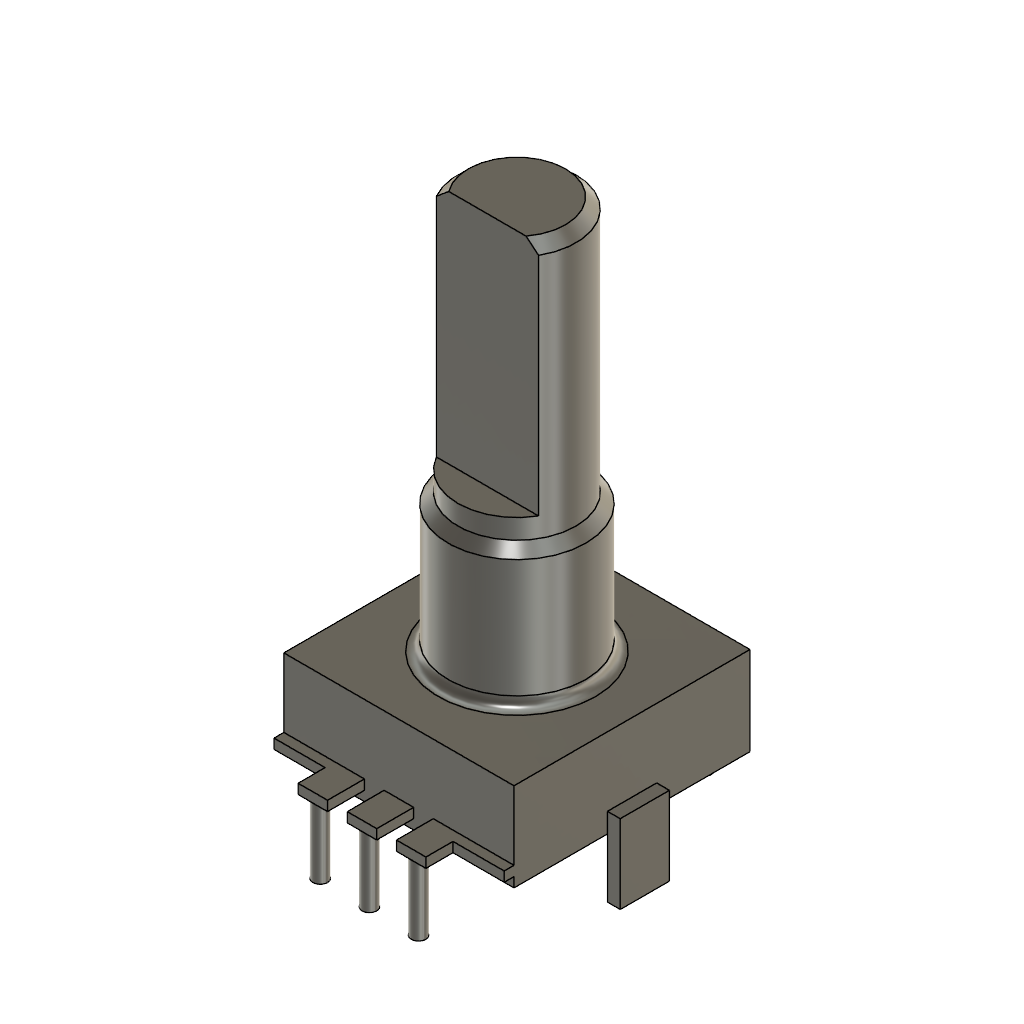
EC11E single rotary (Autodesk Fusion 360 design; units mm, degrees)
Autodesk Fusion 360 part; units mm, degrees
sketch "Skizze1" plane through (0, 0, 0) normal (0, 0, 1) x (1, 0, 0)
  line L0 (0, 0) -> (-11.7, 0)
  line L1 (-11.7, 0) -> (-11.7, 12)
  line L2 (-11.7, 12) -> (0, 12)
  line L3 (0, 12) -> (0, 0)
  dimension "d1" = 11.7
  dimension "d2" = 12
  constraint horizontal L0
  constraint vertical L1
  constraint horizontal L2
  constraint vertical L3
  constraint coincident L0.start L3.end
  measures "d1" distance of L1.end L2.end
  measures "d2" distance of L0.end L1.end
extrude "Extrusion1" add sketch "Skizze1" along normal blind 4.5
ref_plane "Arbeitsebene1" through (0, 0, 0.5) normal (0, 0, 1) x (1, 0, 0)
sketch "Skizze2" plane through (0, 0, 0.5) normal (0, 0, 1) x (1, 0, 0)
  line L0 (0, 12) -> (-11.7, 12)
  line L1 (-11.7, 12) -> (-11.7, 0)
  line L2 (-11.7, 0) -> (0, 0)
  line L3 (0, 0) -> (0, 12)
  line L4 (-8.35, 12) -> (-8.35, 19) construction
  line L5 (-3.35, 12) -> (-3.35, 19) construction
  line L6 (-8.35, 0) -> (-8.35, -5) construction
  line L7 (-5.85, 0) -> (-5.85, -5) construction
  line L8 (-3.35, 0) -> (-3.35, -5) construction
  line L9 (-7.6, 12) -> (-9.1, 12)
  line L10 (-9.1, 12) -> (-9.1, 13.375)
  line L11 (-9.1, 13.375) -> (-7.6, 13.375)
  line L12 (-7.6, 13.375) -> (-7.6, 12)
  line L13 (-2.6, 12) -> (-4.1, 12)
  line L14 (-4.1, 12) -> (-4.1, 13.375)
  line L15 (-4.1, 13.375) -> (-2.6, 13.375)
  line L16 (-2.6, 13.375) -> (-2.6, 12)
  line L17 (-2.6, 0) -> (-4.1, 0)
  line L18 (-4.1, 0) -> (-4.1, -1.875)
  line L19 (-4.1, -1.875) -> (-2.6, -1.875)
  line L20 (-2.6, -1.875) -> (-2.6, 0)
  line L21 (-6.6, 0) -> (-5.1, 0)
  line L22 (-5.1, 0) -> (-5.1, -1.875)
  line L23 (-5.1, -1.875) -> (-6.6, -1.875)
  line L24 (-6.6, -1.875) -> (-6.6, 0)
  line L25 (-9.1, 0) -> (-7.6, 0)
  line L26 (-7.6, 0) -> (-7.6, -1.875)
  line L27 (-7.6, -1.875) -> (-9.1, -1.875)
  line L28 (-9.1, -1.875) -> (-9.1, 0)
  line L29 (-9.1, 0) -> (-11.7, 0)
  line L30 (-11.7, 0) -> (-11.7, -0.5)
  line L31 (-11.7, -0.5) -> (-9.1, -0.5)
  line L32 (-9.1, -0.5) -> (-9.1, 0)
  line L33 (-2.6, 0) -> (0, 0)
  line L34 (0, 0) -> (0, -0.5)
  line L35 (0, -0.5) -> (-2.6, -0.5)
  line L36 (-2.6, -0.5) -> (-2.6, 0)
  circle A0 centre (-8.35, 13) radius 0.375
  circle A1 centre (-3.35, 13) radius 0.375
  circle A2 centre (-8.35, -1.5) radius 0.375
  circle A3 centre (-5.85, -1.5) radius 0.375
  circle A4 centre (-3.35, -1.5) radius 0.375
  line L37 (-11.7, 6) -> (0, 6) construction
  line L38 (-11.7, 7.25) -> (-12.35, 7.25)
  line L39 (-12.35, 7.25) -> (-12.35, 4.75)
  line L40 (-12.35, 4.75) -> (-11.7, 4.75)
  line L41 (-11.7, 4.75) -> (-11.7, 7.25)
  line L42 (0, 7.25) -> (0.65, 7.25)
  line L43 (0.65, 7.25) -> (0.65, 4.75)
  line L44 (0.65, 4.75) -> (0, 4.75)
  line L45 (0, 4.75) -> (0, 7.25)
  line L46 (-11.6, 7.25) -> (-11.6, 4.75)
  line L47 (-0.1, 7.25) -> (-0.1, 4.75)
  dimension "d7" = 5
  dimension "d8" = 5
  dimension "d9" = 1.5
  dimension "d11" = 0.5
  dimension "d12" = 0.75
  dimension "d13" = 0.75
  dimension "d14" = 0.75
  dimension "d15" = 0.75
  dimension "d16" = 0.75
  dimension "d17" = 7
  dimension "d18" = 7
  dimension "d19" = 7.5
  dimension "d20" = 7.5
  dimension "d21" = 7.5
  dimension "d26" = 0.75
  dimension "d27" = 0.75
  dimension "d28" = 13
  dimension "d46" = 2.5
  constraint coincident L0 L4.start
  constraint perpendicular L0 L4
  constraint coincident L0 L5.start
  constraint perpendicular L0 L5
  constraint coincident L2 L6.start
  constraint perpendicular L2 L6
  constraint midpoint L2 L7.start
  constraint perpendicular L2 L7
  constraint coincident L2 L8.start
  constraint perpendicular L2 L8
  constraint horizontal L9
  constraint vertical L10
  constraint horizontal L11
  constraint vertical L12
  constraint coincident L0 L9.start
  constraint horizontal L13
  constraint vertical L14
  constraint horizontal L15
  constraint vertical L16
  constraint coincident L0 L13.start
  constraint horizontal L17
  constraint vertical L18
  constraint horizontal L19
  constraint vertical L20
  constraint coincident L2 L17.start
  constraint horizontal L21
  constraint vertical L22
  constraint horizontal L23
  constraint vertical L24
  constraint coincident L2 L21.start
  constraint horizontal L25
  constraint vertical L26
  constraint horizontal L27
  constraint vertical L28
  constraint coincident L2 L25.start
  constraint symmetric L6.end L7 L8.end
  constraint symmetric L4.end L5.end L7
  constraint symmetric L4 L10 L12
  constraint symmetric L5 L14 L16
  constraint symmetric L7 L22 L24
  constraint equal L10 L14
  constraint equal L11 L15
  constraint equal L11 L27
  constraint equal L23 L27
  constraint equal L19 L23
  constraint horizontal L29
  constraint vertical L30
  constraint horizontal L31
  constraint vertical L32
  constraint horizontal L33
  constraint vertical L34
  constraint horizontal L35
  constraint vertical L36
  constraint equal L30 L34
  constraint coincident L1.end L2.start
  constraint coincident L4 A0.centre
  constraint coincident L5 A1.centre
  constraint coincident L6 A2.centre
  constraint coincident L7 A3.centre
  constraint coincident L8 A4.centre
  constraint midpoint L1 L37.start
  constraint midpoint L3 L37.end
  constraint tangent L11 A0
  constraint tangent L27 A2
  constraint tangent L23 A3
  constraint tangent L19 A4
  constraint horizontal L38
  constraint vertical L39
  constraint horizontal L40
  constraint vertical L41
  constraint coincident L1 L38.start
  constraint horizontal L42
  constraint vertical L43
  constraint horizontal L44
  constraint vertical L45
  constraint coincident L3 L42.start
  constraint symmetric L37 L38 L40
  constraint symmetric L37 L42 L44
  constraint equal L38 L42
  constraint equal L39 L43
  constraint coincident L38 L46.start
  constraint coincident L40 L46.end
  constraint perpendicular L40 L46
  constraint coincident L42 L47.start
  constraint coincident L44 L47.end
  constraint perpendicular L44 L47
  measures "d7" distance of L4 L5
  measures "d8" distance of L6 L8
  measures "d9" distance of L10.end L11.end
  measures "d11" distance of L1.end L30.end
  measures "d12" diameter of A0
  measures "d13" diameter of A1
  measures "d14" diameter of A2
  measures "d15" diameter of A3
  measures "d16" diameter of A4
  measures "d17" distance of A0.centre L37
  measures "d18" distance of A1.centre L37
  measures "d19" distance of A2.centre L37
  measures "d20" distance of A3.centre L37
  measures "d21" distance of A4.centre L37
  measures "d26" distance of L39 L46
  measures "d27" distance of L43 L47
  measures "d28" distance of L39 L43
  measures "d46" distance of L38.end L39.end
extrude "Extrusion2" add sketch "Skizze2" along normal blind 0.5 contours A1 | L0 L13 L14 L15 L16 | L3 L42 L43 L44 L45 | A0 | L0 L9 L10 L11 L12 | L2 L20 L33 L34 L35 L36 | A4 | L2 L17 L18 L19 L20 L36 | L1 L38 L39 L40 L41 | A3 | L2 L21 L22 L23 L24 | L2 L28 L29 L30 L31 L32 | A2 | L2 L25 L26 L27 L28 L32
extrude "Extrusion3" add sketch "Skizze2" against normal blind 3.5 contours A1 | L3 L42 L43 L44 L45 | A0 | A4 | L1 L38 L39 L40 L41 | A3 | A2
ref_plane "Arbeitsebene2" through (0, 6, 0) normal (0, 1, 0) x (0, 0, 1)
sketch "Skizze3" plane through (0, 6, 0) normal (0, 1, 0) x (1, 0, 0)
  line L0 (-4.1, -1) -> (0, -1)
  line L1 (0, -1) -> (0, -4.5)
  line L2 (0, -4.5) -> (-11.7, -4.5)
  line L3 (-11.7, -4.5) -> (-11.7, -1)
  line L4 (-11.7, -1) -> (-7.6, -1)
  line L5 (-7.6, -1) -> (-7.6, -0.5)
  line L6 (-7.6, -0.5) -> (-11.7, -0.5)
  line L7 (-11.7, -0.5) -> (-11.7, 0)
  line L8 (-11.7, 0) -> (0, 0)
  line L9 (0, 0) -> (0, -0.5)
  line L10 (0, -0.5) -> (-4.1, -0.5)
  line L11 (-4.1, -0.5) -> (-4.1, -1)
  line L12 (-5.1, -1) -> (-5.1, -0.5)
  line L13 (-5.1, -0.5) -> (-6.6, -0.5)
  line L14 (-6.6, -0.5) -> (-6.6, -1)
  line L15 (-6.6, -1) -> (-5.1, -1)
  line L16 (-5.85, -4.5) -> (-5.85, -18.5)
  line L17 (-5.85, -4.5) -> (-1.85, -4.5)
  line L18 (-2.35, -5) -> (-2.35, -11)
  arc A0 (-1.85, -4.5) -> (-2.35, -5) centre (-1.85, -5) ccw
  line L19 (-2.35, -11) -> (-2.85, -11.5)
  line L20 (-2.85, -11.5) -> (-2.85, -23.9697)
  line L21 (-2.85, -23.9697) -> (-3.3803, -24.5)
  line L22 (-3.3803, -24.5) -> (-5.85, -24.5)
  line L23 (-5.85, -24.5) -> (-5.85, -4.5)
  dimension "d31" = 1
  dimension "d32" = 7
  dimension "d33" = 6
  dimension "d34" = 135
  dimension "d35" = 135
  dimension "d36" = 7
  dimension "d40" = 0.75
  dimension "d41" = 20
  constraint midpoint L2 L16.start
  constraint perpendicular L2 L16
  constraint tangent L17 A0
  constraint vertical L18
  constraint tangent L18 A0
  constraint parallel L18 L20
  constraint coincident L16 L22.end
  constraint perpendicular L16 L22
  constraint horizontal L17
  measures "d31" diameter of A0
  measures "d34" angle of L18 L19
  measures "d35" angle of L20 L21
  measures "d36" distance of L17 L19.end
  measures "d40" distance of L20.end L21.end
  measures "d41" distance of L2 L22
revolve "Drehen1" add sketch "Skizze3" angle 360 about axis through (-5.85, 6, 4.5) along (0, 0, 1) contours L2 L16 L17 L18 A0 L19 L20 L21 L22 L23
sketch "Skizze4" plane through (0, 0, 24.5) normal (0, 0, 1) x (-1, 0, 0)
  circle A0 centre (5.85, -6) radius 2.4697
  circle A1 centre (5.85, -6) radius 3
  line L0 (8.4481, -4.5) -> (3.2519, -4.5)
  arc A2 (8.4481, -4.5) -> (3.2519, -4.5) centre (5.85, -6) ccw
  line L1 (5.85, -4.5) -> (5.85, -9) construction
  dimension "d43" = 4.5
  constraint coincident A1 L0.start
  constraint coincident A1 L0.end
  constraint horizontal L0
  constraint concentric A1 A2
  constraint midpoint L0 L1.start
  constraint coincident A1 L1.end
  constraint perpendicular A1 L1
  measures "d43" distance of L1.start L1.end
extrude "Extrusion4" cut sketch "Skizze4" against normal blind 12 contours A0 L0 | A0 A1 L0 A2 picked at (5.6769, -4.1952)
equation "d13 = d12"
equation "d14 = d12"
equation "d15 = d12"
equation "d16 = d12"
